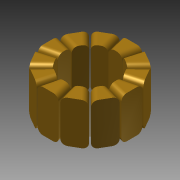
# Autodesk Inventor part: coils
Saved by Autodesk Inventor 2012 (Build 160160000, 160)
## iProperties
Created: 2014-07-09
Part Number: coils
Material: Default
Document SubType Name: Modeling
Designer: Anon
Density: 1 g/cm^3
Author: Anon
Autodesk Inventor part; units mm, degrees
ref_plane "YZ Plane" through (0, 0, 0) normal (1, 0, 0) x (0, 1, 0)
ref_plane "XZ Plane" through (0, 0, 0) normal (0, 1, 0) x (-1, 0, 0)
ref_plane "XY Plane" through (0, 0, 0) normal (0, 0, 1) x (1, 0, 0)
sketch "Sketch1" plane through (0, 0, 0) normal (0, 0, 1) x (1, 0, 0)
  line L0 (-2, 8) -> (2, 8)
  line L1 (2, 8) -> (3.25, 13)
  line L2 (3.25, 13) -> (-3.25, 13)
  line L3 (-3.25, 13) -> (-2, 8)
  point P0 (0, 0)
  dimension "d0" = 8
  dimension "d1" = 5
  dimension "d2" = 4
  dimension "d3" = 2
  dimension "d4" = 6.5
  dimension "d5" = 3.25
  constraints: 8 end point, 1 horizontal, 1 parallel
  measures "d0" distance from line of point (0, 0) L0
  measures "d1" distance between parallel lines of L2 L0
  measures "d2" distance of L0.end L0.start
  measures "d3" horizontal distance of L0.start point (0, 0)
  measures "d4" distance of L1.end L2.end
  measures "d5" horizontal distance of point (0, 0) L1.end
extrude "Extrusion1" add sketch "Sketch1" along normal blind 13
fillet "Fillet1" radius 1.6 4 edges at (2.625, 10.5, 13) (-2.625, 10.5, 13) (2.625, 10.5, 0) (-2.625, 10.5, 0)
pattern_circular "Circular Pattern1" count 12 over 360 about axis through (0, 0, -10) along (0, 0, 1) of "Extrusion1", "Fillet1"
body "Solid1"
